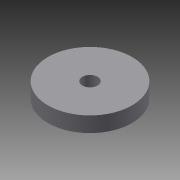
# Autodesk Inventor part: tiedown-hook-mount
Saved by Autodesk Inventor 2015 (Build 190159000, 159)
## iProperties
Created: 2015-02-01
Part Number: tiedown-hook-mount
Material: Generic
Document SubType Name: Modeling
Designer: bovine
Density: 1 g/cm^3
Appearance: Default
Author: bovine
Autodesk Inventor part; units mm, degrees
ref_plane "YZ Plane" through (0, 0, 0) normal (1, 0, 0) x (0, 1, 0)
ref_plane "XZ Plane" through (0, 0, 0) normal (0, 1, 0) x (-1, 0, 0)
ref_plane "XY Plane" through (0, 0, 0) normal (0, 0, 1) x (1, 0, 0)
sketch "SketchCircles" plane through (0, 0, 0) normal (0, 1, 0) x (-1, 0, 0)
  circle A0 centre (0, 0) radius 12.7
  circle A1 centre (0, 0) radius 6.35
  circle A2 centre (0, 0) radius 17.4625
  dimension "d0" = 25.4
  dimension "d1" = 12.7
  dimension "d2" = 34.925
  constraints: 3 centre point, 3 coincident
  measures "d0" diameter of A0
  measures "d1" diameter of A1
  measures "d2" diameter of A2
extrude "Extrusion100" add sketch "SketchCircles" along normal blind 6.35 contours A0 | A1 | A2
sketch "SketchLines" plane through (0, 0, 0) normal (0, -1, 0) x (1, 0, 0)
  line L0 (-17.7365, 0) -> (17.5532, 0)
  line L1 (-0.0917, 17.7823) -> (-0.0917, -17.324)
  point P0 (0, 0)
  constraints: 4 end point, 1 horizontal, 1 vertical
hole "Hole1" at (0, 0, 0) direction (0, 1, 0) diameter 25.4 depth 3.175
sketch "Sketch3" plane through (0, 3.175, 0) normal (0, -1, 0) x (1, 0, 0)
  circle A0 centre (0, 0) radius 6.35
  dimension "d12" = 12.7
  constraints: 1 centre point, 1 coincident
  measures "d12" diameter of A0
extrude "Extrusion2" add sketch "Sketch3" along normal blind 3.175
chamfer "Chamfer1" distance 1.397 angle 45 1 edges at (0, 0, 12.7)
chamfer "Chamfer2" distance 1.397 angle 45 1 edges at (-6.35, 0, 0)
sketch "Sketch4" plane through (0, 6.35, 0) normal (0, 1, 0) x (1, 0, 0)
  circle A0 centre (0, 0) radius 3.9688
  dimension "d21" = 7.9375
  constraints: 1 centre point, 1 coincident
  measures "d21" diameter of A0
hole "Hole2" at (0, 6.35, 0) direction (0, -1, 0) diameter 6.35 depth 12.7
body "Solid1"
